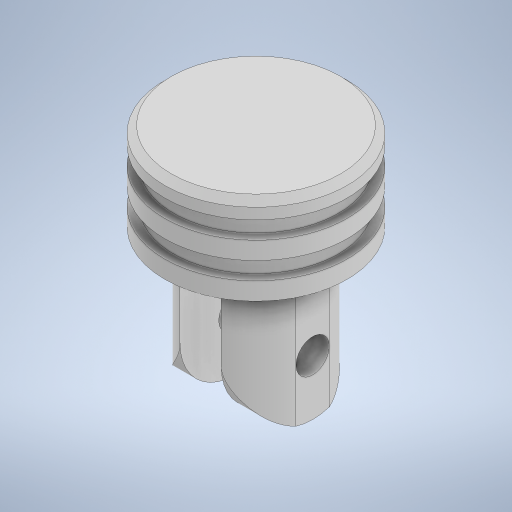
# Autodesk Inventor part: Piston
Saved by Autodesk Inventor 2023 (Build 270158000, 158)
## iProperties
Created: 2022-12-22
Part Number: Piston
Material: Generic
Document SubType Name: Modeling
Designer: tgr41
Density: 1 g/cm^3
Appearance: Default
Author: tgr41
Autodesk Inventor part; units mm, degrees
ref_plane "YZ Plane" through (0, 0, 0) normal (1, 0, 0) x (0, 1, 0)
ref_plane "XZ Plane" through (0, 0, 0) normal (0, 1, 0) x (-1, 0, 0)
ref_plane "XY Plane" through (0, 0, 0) normal (0, 0, 1) x (1, 0, 0)
sketch "Sketch1" plane through (0, 0, 0) normal (1, 0, 0) x (0, 1, 0)
  line L0 (0, 0) -> (0, -17.3736)
  line L1 (0, -17.3736) -> (3.3528, -17.3736)
  line L2 (3.3528, -17.3736) -> (3.3528, -15.6972)
  line L3 (3.3528, -15.6972) -> (6.7056, -15.6972)
  line L4 (6.7056, -15.6972) -> (6.7056, -17.3736)
  line L5 (6.7056, -17.3736) -> (10.0584, -17.3736)
  line L6 (10.0584, -17.3736) -> (10.0584, -15.6972)
  line L7 (10.0584, -15.6972) -> (13.4112, -15.6972)
  line L8 (13.4112, -15.6972) -> (13.4112, -17.3736)
  line L9 (13.4112, -17.3736) -> (16.764, -17.3736)
  line L10 (16.764, -17.3736) -> (16.764, 0)
  line L11 (16.764, 0) -> (0, 0)
  dimension "d0" = 17.3736
  dimension "d1" = 3.3528
  dimension "d2" = 1.6764
  dimension "d3" = 3.3528
  dimension "d4" = 1.6764
  dimension "d5" = 3.3528
  dimension "d6" = 1.6764
  dimension "d7" = 3.3528
  dimension "d8" = 1.6764
  dimension "d9" = 3.3528
  constraints: 24 end point, 6 perpendicular, 4 point on line, 1 horizontal, 1 vertical
  measures "d0" distance of L0.start L0.end
  measures "d1" distance of L0.end L1.end
  measures "d2" distance of L1.end L2.end
  measures "d3" distance of L2.end L3.end
  measures "d4" distance of L3.end L4.end
  measures "d5" distance of L4.end L5.end
  measures "d6" distance of L5.end L6.end
  measures "d7" distance of L6.end L7.end
  measures "d8" distance of L7.end L8.end
  measures "d9" distance of L8.end L9.end
revolve "Revolution1" add sketch "Sketch1" angle 360 about axis through (0, 16.764, 0) along (0, -1, 0)
sketch "Sketch2" plane through (0, 0, 0) normal (0, -1, 0) x (1, 0, 0)
  line L0 (3.937, 16.9216) -> (3.937, -16.9216)
  line L1 (10.795, 13.6129) -> (10.795, -13.6129)
  circle A0 centre (0, 0) radius 17.3736
  line L2 (-3.937, 16.9216) -> (-3.937, -16.9216)
  line L3 (-10.795, 13.6129) -> (-10.795, -13.6129)
  line L4 (10.795, 0) -> (10.795, 3.175)
  circle A1 centre (0, 0) radius 11.2522
  point P0 (-10.795, -3.175)
  point P1 (-3.937, -10.541)
  point P2 (-3.937, 10.541)
  point P3 (-10.795, 3.175)
  point P4 (3.937, -10.541)
  point P5 (10.795, -3.175)
  point P6 (3.937, 10.541)
  dimension "d18" = 3.175
  constraints: 10 end point, 2 coincident, 2 point on circle, 1 centre point, 1 midpoint, 1 point on line, 3 other
  measures "d18" distance of L4.start L4.end
extrude "Extrusion2" add sketch "Sketch2" along normal blind 31.75 contours A1 L1 L0 | L2 A1 L3
chamfer "Chamfer1" distance 1.27 angle 45 1 edges at (0, 16.764, 17.3736)
fillet "Fillet1" radius 3.175 6 edges at (-8.2354, 0, 7.6675) (-10.795, 0, 0) (-8.2354, 0, -7.6675) (8.2354, 0, -7.6675) (10.795, 0, 0) (8.2354, 0, 7.6675)
sketch "Sketch3" plane through (-10.795, -31.75, -3.175) normal (-1, 0, 0) x (0, 0, 1)
  line L0 (3.175, 31.75) -> (3.175, -0.2672)
  line L1 (-7.366, 0) -> (13.716, 0) projected
  line L2 (3.175, 0) -> (3.175, 31.75)
  line L3 (17.0547, 31.75) -> (-10.7047, 31.75) projected
  circle A0 centre (3.175, 15.875) radius 3.175
  line L4 (6.35, 28.575) -> (6.35, 0) projected
  line L5 (13.716, 28.575) -> (13.716, 0) projected
  line L6 (13.716, 15.875) -> (21.6124, 15.7414)
  line L7 (21.6124, 15.7414) -> (21.6124, -6.9282)
  line L8 (21.6124, -6.9282) -> (-12.8487, -6.9282)
  line L9 (-12.8487, -6.9282) -> (-12.8487, 16.3244)
  line L10 (-12.8487, 16.3244) -> (-7.366, 15.875)
  line L11 (-7.366, 28.575) -> (-7.366, 0) projected
  arc A1 (-7.366, 15.875) -> (13.716, 15.875) centre (3.175, 15.875) ccw
  constraints: 14 end point, 3 perpendicular, 3 point on line, 2 centre point, 2 midpoint, 2 point on circle, 2 tangent, 2 vertical, 1 coincident
extrude "Extrusion3" cut sketch "Sketch3" against normal blind 31.75 contours A0 L0 | L0 A0 | A1 L4 L1 L0 | L0 L1 L11 A1 | A1 L5 L1 L4 | L1 L5 L6 L7 L8 L9 L10 L11
body "Solid1"
